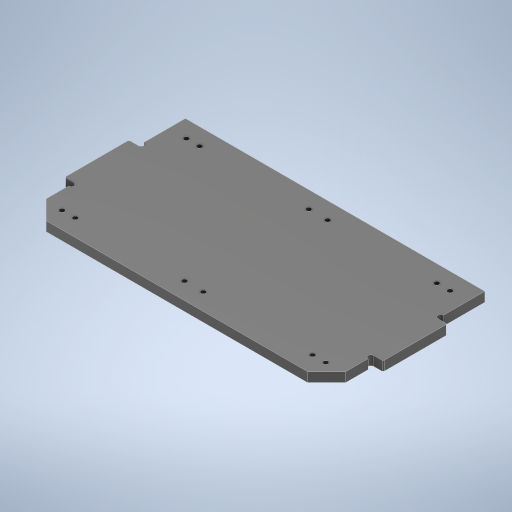
# Autodesk Inventor part: TorsoElectronicBoxBoardMountFrame
Saved by Autodesk Inventor 2024.2 (Build 282272000, 272)
## iProperties
Created: 2024-01-11
Part Number: TorsoElectronicBoxBoardMountFrame
Material: Acetal Resin, Black
Document SubType Name: Modeling
Designer: Masato Kubotera
Density: 1.425 g/cm^3
Appearance: Smooth - Black
Vendor: meviy
Mass: 41.0153 g
Surface Area: 171.301 cm^2
Volume: 28.7827 cm^3
Author: Masato Kubotera
Autodesk Inventor part; units mm, degrees
ref_plane "YZ Plane" through (0, 0, 0) normal (1, 0, 0) x (0, 1, 0)
ref_plane "XZ Plane" through (0, 0, 0) normal (0, 1, 0) x (-1, 0, 0)
ref_plane "XY Plane" through (0, 0, 0) normal (0, 0, 1) x (1, 0, 0)
sketch "Sketch1" plane through (0, 0, 0) normal (0, 0, 1) x (1, 0, 0)
  line L0 (-42, -79.5) -> (42, -79.5)
  line L1 (42, -79.5) -> (42, 79.5)
  line L2 (42, 79.5) -> (-42, 79.5) construction
  line L3 (-42, 79.5) -> (-42, -79.5)
  line L4 (-42, -79.5) -> (42, 79.5) construction
  line L5 (42, -79.5) -> (-42, 79.5) construction
  line L6 (-42, 0) -> (42, 0)
  line L7 (-17, 84.5) -> (17, 84.5)
  line L8 (17, 84.5) -> (17, 79.5)
  line L9 (-17, 84.5) -> (-17, 79.5)
  arc A0 (-20, 79.5) -> (-17, 79.5) centre (-18.5, 79.5) ccw
  line L10 (-23, 79.5) -> (-23, 73.5) construction
  line L11 (17, 84.5) -> (17, 79.5)
  arc A1 (17, 79.5) -> (20, 79.5) centre (18.5, 79.5) ccw
  line L12 (23, 79.5) -> (23, 73.5) construction
  line L13 (0, 79.5) -> (0, 84.5) construction
  line L14 (-33, -70) -> (33, -70) construction
  line L15 (33, -70) -> (33, 70) construction
  line L16 (33, 70) -> (-33, 70) construction
  line L17 (-33, 70) -> (-33, -70) construction
  line L18 (-33, -70) -> (33, 70) construction
  line L19 (33, -70) -> (-33, 70) construction
  line L20 (0, -70) -> (0, 70) construction
  line L21 (-33, 5) -> (33, 5) construction
  line L22 (33, 5) -> (33, 63) construction
  line L23 (33, 63) -> (-33, 63) construction
  line L24 (-33, 63) -> (-33, 5) construction
  line L25 (-33, 5) -> (33, 63) construction
  line L26 (33, 5) -> (-33, 63) construction
  line L27 (-40, 1.5) -> (40, 1.5) construction
  line L28 (40, 1.5) -> (40, 66.5) construction
  line L29 (40, 66.5) -> (-40, 66.5) construction
  line L30 (-40, 66.5) -> (-40, 1.5) construction
  line L31 (-40, 1.5) -> (40, 66.5) construction
  line L32 (40, 1.5) -> (-40, 66.5) construction
  line L33 (33, -70) -> (-33, -70) construction
  line L34 (-40, 34) -> (40, 34) construction
  line L35 (-34, 74.5) -> (34, 74.5)
  line L36 (-30, 5) -> (-30, 3.5)
  arc A2 (-30, 5) -> (-32.75, 7.9896) centre (-33, 5) ccw
  line L37 (-28, 1.5) -> (28, 1.5)
  line L38 (30, 5) -> (30, 3.5)
  arc A3 (33.6, 7.9394) -> (30, 5) centre (33, 5) ccw
  arc A4 (-30, 3.5) -> (-28, 1.5) centre (-28, 3.5) ccw
  arc A5 (36, 72.5) -> (34, 74.5) centre (34, 72.5) ccw
  arc A6 (33.6, 7.9394) -> (36, 9.899) centre (34, 9.899) ccw
  arc A7 (28, 1.5) -> (30, 3.5) centre (28, 3.5) ccw
  line L39 (-42, 79.5) -> (-20, 79.5)
  line L40 (20, 79.5) -> (42, 79.5)
  arc A8 (33.6, 72.9394) -> (33.6, 67.0606) centre (33, 70) ccw
  arc A9 (33.6, 65.9394) -> (33.6, 60.0606) centre (33, 63) ccw
  line L41 (36, 67.899) -> (36, 72.5)
  line L42 (36, 74.899) -> (36, 58.101)
  line L43 (36, 65.101) -> (36, 9.899)
  arc A10 (36, 65.101) -> (33.6, 67.0606) centre (34, 65.101) ccw
  arc A11 (33.6, 72.9394) -> (36, 74.899) centre (34, 74.899) ccw
  arc A12 (36, 58.101) -> (33.6, 60.0606) centre (34, 58.101) ccw
  arc A13 (33.6, 65.9394) -> (36, 67.899) centre (34, 67.899) ccw
  arc A14 (-30, 5) -> (-33.6, 7.9394) centre (-33, 5) ccw
  line L44 (-30, 5) -> (-30, 3.5)
  arc A15 (-34, 74.5) -> (-36, 72.5) centre (-34, 72.5) ccw
  arc A16 (-36, 9.899) -> (-33.6, 7.9394) centre (-34, 9.899) ccw
  arc A17 (-30, 3.5) -> (-28, 1.5) centre (-28, 3.5) ccw
  arc A18 (-33.6, 67.0606) -> (-33.6, 72.9394) centre (-33, 70) ccw
  line L45 (-36, 67.899) -> (-36, 72.5)
  line L46 (-36, 74.899) -> (-36, 58.101)
  line L47 (-36, 65.101) -> (-36, 9.899)
  arc A19 (-33.6, 67.0606) -> (-36, 65.101) centre (-34, 65.101) ccw
  arc A20 (-36, 74.899) -> (-33.6, 72.9394) centre (-34, 74.899) ccw
  arc A21 (-33.6, 60.0606) -> (-36, 58.101) centre (-34, 58.101) ccw
  arc A22 (-36, 67.899) -> (-33.6, 65.9394) centre (-34, 67.899) ccw
  arc A23 (-33.6, 60.0606) -> (-33.6, 65.9394) centre (-33, 63) ccw
  point P0 (0, 0)
  point P1 (0, 0)
  point P2 (33, -70)
  point P3 (0, 34)
  point P4 (0, -34)
  point P5 (0, -34)
  point P6 (-29.66, 74.5)
  point P7 (29.66, 74.5)
  point P8 (-30, 1.5)
  point P9 (30, 1.5)
  point P10 (36, 70)
  point P11 (36, 70)
  point P12 (36, 63)
  point P13 (36, 63)
  point P14 (-32.75, 7.9896)
  point P15 (36, 70.1995)
  point P16 (-35.4293, 66.5)
  point P17 (-35.6004, 73.6995)
  point P18 (35.4293, 66.5)
  point P19 (35.6004, 73.6995)
  dimension "d1" = 159
  dimension "d2" = 1.5
  dimension "d3" = 5
  dimension "d5" = 6
  dimension "d6" = 6
  dimension "d36" = 25
  dimension "d40" = 66
  dimension "d41" = 140
  dimension "d42" = 58
  dimension "d43" = 66
  dimension "d44" = 80
  dimension "d45" = 65
  dimension "d67" = 5
  dimension "d68" = 2
  dimension "d70" = 42
  dimension "d71" = 84
  dimension "d73" = 25
  dimension "d75" = 10
  dimension "d76" = 6
  dimension "d77" = 2
  dimension "d78" = 3
  dimension "d87" = 6
  constraints: 96 end point, 52 point on circle, 29 symmetric about line, 24 centre point, 19 midpoint, 17 tangent, 16 point on line, 13 coincident, 8 parallel, 7 equal radius, 7 horizontal, 7 vertical, 4 collinear, 4 perpendicular, 14 other
  measures "d1" distance of L1.end L0.end
  measures "d2" radius of A0
  measures "d3" distance of L7.start L9.end
  measures "d5" distance of L10.start L10.end
  measures "d6" distance between parallel lines of L9 L10
  measures "d36" distance between parallel lines of L8 L1
  measures "d40" distance of L15.end L16.end
  measures "d41" distance of L14.end L15.end
  measures "d42" distance of L23.end L21.start
  measures "d43" distance of L22.end L23.end
  measures "d44" distance of L29.end L28.end
  measures "d45" distance of L27.end L28.end
  measures "d67" distance between parallel lines of L2 L35
  measures "d68" radius of A4
  measures "d70" distance between parallel lines of L1 L20
  measures "d71" distance between parallel lines of L1 L3
  measures "d73" distance between parallel lines of L9 L3
  measures "d75" diameter of point (-33, 5) L6
  measures "d76" diameter of A9
  measures "d77" radius of A10
  measures "d78" diameter of L37 L6
  measures "d87" distance from line of L1 point (36, 70.199)
extrude "Extrusion1" add sketch "Sketch1" along normal blind 5 contours L3 L39 A0 L9 L7 L8 A1 L40 L1 L6 | L35 A5 A11 A8 A10 A13 A9 A12 L43 A6 A3 L38 A7 L37 A4 L36 A2 A14 A16 L47 A21 A23 A22 A19 A18 A20 A15 | A20 A18 A19 A22 L45 A15 | A15 L46 A20 | A11 L42 A5 | A5 L41 A13 A10 A8 A11 | A22 A19 L46 | L42 A10 A13 | A19 A22 A23 A21 L46 | L42 A12 A9 A13 A10
chamfer "Chamfer1" distance 0.5 angle 45 2 edges at (17, 84.5, 2.5) (-17, 84.5, 2.5)
chamfer "Chamfer2" distance 10 angle 45 1 edges at (42, 79.5, 2.5)
sketch "Sketch4" plane through (20, 79.5, 5) normal (0, 1, 0) x (1, 0, 0)
  line L0 (12, 5) -> (0, 5) projected
  line L1 (3, 5) -> (3, 0)
  line L2 (12, 0) -> (0, 0) projected
  line L3 (-40, 5) -> (-62, 5) projected
  line L4 (-43, 5) -> (-43, 0)
  line L5 (-40, 0) -> (-62, 0) projected
  point P0 (-20, 5)
  point P1 (-52, 5)
  point P2 (-52, 0)
  point P3 (3, 5)
  point P4 (3, 2.5)
  point P5 (-43, 2.5)
  constraints: 4 end point, 2 midpoint, 2 point on line, 2 vertical
hole "Side-M2" [suppressed]
hole "M3" at (-33, -70, 0) at (33, -70, 0) at (33, 70, 0) at (-33, 70, 0) at (-33, 5, 0) at (-33, 63, 0) at (33, 5, 0) at (33, 63, 0) direction (0, 0, 1) diameter 2.459 end through all thread size "M3x0.5" class "6H" standard "ANSI Metric M Profile"
mirror "Mirror1" about plane through (0, 0, 0) normal (0, 1, 0)
body "Solid1"
